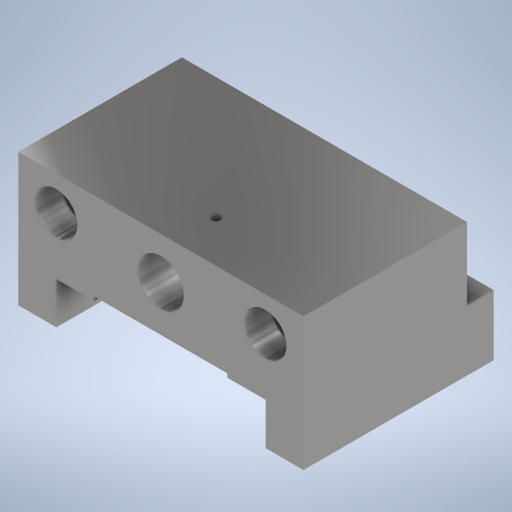
# Autodesk Inventor part: lose back
Saved by Autodesk Inventor 2023.2 (Build 272271000, 271)
## iProperties
Created: 2023-02-02
Part Number: lose back
Material: Steel, Mild
Document SubType Name: Modeling
Designer: Aditya
Density: 7.85 g/cm^3
Appearance: Semi-Polished
Author: Aditya
Autodesk Inventor part; units mm, degrees
ref_plane "YZ Plane" through (0, 0, 0) normal (1, 0, 0) x (0, 1, 0)
ref_plane "XZ Plane" through (0, 0, 0) normal (0, 1, 0) x (-1, 0, 0)
ref_plane "XY Plane" through (0, 0, 0) normal (0, 0, 1) x (1, 0, 0)
sketch "Sketch1" plane through (0, 0, 0) normal (0, 0, 1) x (1, 0, 0)
  line L0 (75, 0) -> (75, 35)
  line L1 (75, 35) -> (0, 35)
  line L2 (0, 35) -> (0, 0)
  line L3 (0, 0) -> (10, 0)
  line L4 (10, 0) -> (10, 11)
  line L5 (10, 11) -> (20, 11)
  line L6 (20, 11) -> (20, 12)
  line L7 (20, 12) -> (55, 12)
  line L8 (55, 12) -> (55, 11)
  line L9 (55, 11) -> (65, 11)
  line L10 (65, 11) -> (65, 0)
  line L11 (65, 0) -> (75, 0)
  dimension "d0" = 75
  dimension "d1" = 35
  dimension "d2" = 10
  dimension "d3" = 11
  dimension "d4" = 10
  dimension "d5" = 90
  dimension "d6" = 1
  dimension "d7" = 35
  dimension "d8" = 10
  dimension "d9" = 11
  constraints: 24 end point, 6 perpendicular, 2 point on line, 1 horizontal, 1 parallel, 1 vertical
  measures "d0" distance of L1.end L0.end
  measures "d1" distance of L0.end L0.start
  measures "d2" distance of L2.end L3.end
  measures "d3" distance of L3.end L4.end
  measures "d4" distance of L4.end L5.end
  measures "d5" angle of L4 L5
  measures "d6" distance of L5.end L6.end
  measures "d7" distance of L6.end L7.end
  measures "d8" distance of L8.end L9.end
  measures "d9" distance of L9.end L10.end
extrude "Extrusion1" add sketch "Sketch1" along normal blind 50
sketch "Sketch2" plane through (75, 0, 0) normal (1, 0, 0) x (0, 0, -1)
  line L0 (0, 35) -> (-50, 35) projected
  line L1 (0, 35) -> (-7, 35)
  line L2 (-7, 35) -> (-7, 16)
  line L3 (-7, 16) -> (0, 16)
  line L4 (0, 16) -> (0, 35)
  point P0 (0, 0)
  dimension "d12" = 7
  dimension "d13" = 19
  constraints: 8 end point, 2 parallel, 1 horizontal, 1 perpendicular
  measures "d12" distance of L3.end L2.end
  measures "d13" distance of L2.end L1.end
extrude "Extrusion2" cut sketch "Sketch2" against normal through all
sketch "Sketch3" plane through (0, 0, 50) normal (0, 0, 1) x (1, 0, 0)
  line L0 (0, 0) -> (10, 0) projected
  line L1 (65, 0) -> (75, 0) projected
  line L2 (75, 0) -> (75, 35) projected
  line L3 (0, 35) -> (0, 0) projected
  point P0 (10, 26)
  point P1 (65, 26)
  dimension "d16" = 26
  dimension "d17" = 26
  dimension "d18" = 10
  dimension "d19" = 10
  measures "d16" distance from line of L0 point (10, 26)
  measures "d17" distance from line of L1 point (65, 26)
  measures "d18" distance from line of L2 point (65, 26)
  measures "d19" distance from line of L3 point (10, 26)
hole "Hole1" at (10, 26, 50) at (65, 26, 50) direction (0, 0, -1) diameter 6.4 end through all counterbore diameter 11 counterbore depth 7
sketch "Sketch4" plane through (0, 0, 50) normal (0, 0, 1) x (1, 0, 0)
  line L0 (65, 0) -> (75, 0) projected
  line L1 (75, 0) -> (75, 35) projected
  point P0 (0, 0)
  point P1 (37.5, 24)
  dimension "d27" = 24
  dimension "d28" = 37.5
  measures "d27" distance from line of L0 point (37.5, 24)
  measures "d28" distance from line of L1 point (37.5, 24)
hole "Hole2" at (37.5, 24, 50) direction (0, 0, -1) diameter 12 depth 20
sketch "Sketch5" plane through (0, 35, 50) normal (0, 1, 0) x (1, 0, 0)
  line L0 (75, 43) -> (75, 0) projected
  line L1 (75, 0) -> (0, 0) projected
  point P0 (0, 50)
  point P1 (41, 11)
  dimension "d36" = 34
  dimension "d44" = 11
  measures "d36" distance from line of L0 point (41, 11)
  measures "d44" distance from line of L1 point (41, 11)
hole "Hole3" at (41, 35, 39) direction (0, -1, 0) diameter 2.459 depth 8.8 thread size "M3x0.5" class "6H" standard "ISO Metric profile"
sketch "Sketch6" plane through (0, 0, 0) normal (0, -1, 0) x (1, 0, 0)
  line L0 (75, 0) -> (75, 50) projected
  line L1 (0, 0) -> (0, 50) projected
  line L2 (0, 50) -> (10, 50) projected
  line L3 (0, 0) -> (10, 0) projected
  line L4 (65, 50) -> (75, 50) projected
  point P0 (5, 43)
  point P1 (5, 7)
  point P2 (70, 43)
  point P3 (70, 7)
  dimension "d45" = 5
  dimension "d46" = 5
  dimension "d47" = 5
  dimension "d48" = 5
  dimension "d50" = 7
  dimension "d51" = 7
  dimension "d52" = 7
  dimension "d60" = 36
  measures "d45" distance from line of L0 point (70, 7)
  measures "d46" distance from line of L0 point (70, 43)
  measures "d47" distance from line of L1 point (5, 7)
  measures "d48" distance from line of L1 point (5, 43)
  measures "d50" distance from line of L2 point (5, 43)
  measures "d51" distance from line of L3 point (5, 7)
  measures "d52" distance from line of L4 point (70, 43)
  measures "d60" distance of point (70, 7) point (70, 43)
hole "Hole4" at (5, 0, 43) at (5, 0, 7) at (70, 0, 43) at (70, 0, 7) direction (0, 1, 0) diameter 4.134 depth 14.2 thread size "M5x0.8" class "6H" standard "ISO Metric profile"
body "Solid1"
